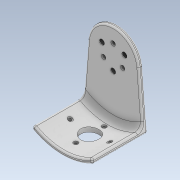
# Autodesk Inventor part: thigh_hip_connector
Saved by Autodesk Inventor 2020 (Build 240168000, 168)
## iProperties
Created: 2021-01-06
Part Number: thigh_hip_connector
Material: Generic
Document SubType Name: Modeling
Designer: DELL
Density: 1 g/cm^3
Appearance: Clear - Blue
Author: DELL
Autodesk Inventor part; units mm, degrees
ref_plane "YZ Plane" through (0, 0, 0) normal (1, 0, 0) x (0, 1, 0)
ref_plane "XZ Plane" through (0, 0, 0) normal (0, 1, 0) x (-1, 0, 0)
ref_plane "XY Plane" through (0, 0, 0) normal (0, 0, 1) x (1, 0, 0)
sketch "Sketch1" plane through (0, 0, 0) normal (0, 0, 1) x (1, 0, 0)
  circle A0 centre (0, 0) radius 22.5
  line L0 (-22.4222, 1.869) -> (-26.5, -47.0505)
  line L1 (22.4222, 1.869) -> (26.5, -47.0505)
  line L2 (9.9593, -5.75) -> (0, 0) construction
  circle A1 centre (8.4134, -4.8575) radius 2
  line L3 (0, 0) -> (9.9593, 5.75) construction
  line L4 (0, 0) -> (-9.9593, -5.75) construction
  circle A2 centre (-8.4134, -4.8575) radius 2
  circle A3 centre (0, 0) radius 9.715 construction
  circle A4 centre (0, 0) radius 11.5 construction
  circle A5 centre (0, 9.715) radius 2
  line L5 (0, 0) -> (-9.9593, 5.75) construction
  line L6 (11.5, 0) -> (-11.5, 0) construction
  circle A6 centre (-9.9593, 5.75) radius 3.75
  circle A7 centre (-9.9593, 5.75) radius 2.25
  line L7 (0, -48.5721) -> (0, 22.5) construction
  circle A8 centre (0, -11.5) radius 2.25
  circle A9 centre (0, -11.5) radius 3.75
  circle A10 centre (9.9593, 5.75) radius 3.75
  circle A11 centre (9.9593, 5.75) radius 2.25
  arc A12 (-26.1314, -42.6281) -> (26.1314, -42.6281) centre (0, 0) ccw
  arc A13 (-26.5, -47.0505) -> (26.5, -47.0505) centre (0, 0) ccw
  point P0 (0, 11.4686)
  point P1 (0, 11.4686)
  point P2 (11.5, 0)
  point P3 (-11.5, 0)
  dimension "d18" = 23
  dimension "d0" = 45
  dimension "d17" = 19.43
  dimension "d19" = 30
  dimension "d20" = 30
  dimension "d21" = 4.5
  dimension "d22" = 7.5
  dimension "d23" = 4
  dimension "d24" = 100
  dimension "d25" = 108
  dimension "d48" = 53
  constraints: 14 end point, 13 centre point, 10 coincident, 9 point on circle, 8 point on line, 6 equal radius, 2 tangent, 1 vertical, 17 other
  measures "d0" diameter of A0
  measures "d17" diameter of A3
  measures "d19" angle to the sketch x axis of L5
  measures "d20" angle to the sketch x axis of L4
  measures "d21" diameter of A11
  measures "d22" diameter of A10
  measures "d23" diameter of A5
  measures "d24" diameter of A12
  measures "d25" diameter of A13
  measures "d48" distance of L1.end L0.end
extrude "Extrusion1" add sketch "Sketch1" along normal blind 4 contours A0 | A0 L1 A12 L0 | L1 A13 L0 A12 | A1 | A2 | A5 | A6 | A9 | A10
extrude "Extrusion2" cut sketch "Sketch1" along normal blind 3.5 contours A6 | A9 | A10 | A11
extrude "Extrusion3" cut sketch "Sketch1" against normal blind 5 from surface at 4 contours A1 | A2 | A5
extrude "Extrusion4" add sketch "Sketch1" along normal blind 45 from surface at 4 contours L1 A13 L0 A12
fillet "Fillet1" radius 5 1 edges at (0, -50, 4)
fillet "Fillet2" radius 1.5 17 edges at (0, -54, 0) (0, -54, 49) (26.5, -47.0505, 24.5) (-26.5, -47.0505, 24.5) (-24.4611, -22.5907, 0) (24.4611, -22.5907, 0) (0, 22.5, 0) (-24.0409, -17.5492, 4) (-25.9834, -40.8531, 5.3489) (-26.1314, -42.6281, 29) (24.0409, -17.5492, 4) (25.9834, -40.8531, 5.3489) (26.1314, -42.6281, 29) (0, 22.5, 4) (0, -50, 49) (-26.3157, -44.8393, 49) (26.3157, -44.8393, 49)
sketch "Sketch2" plane through (0, 0, 0) normal (0, 1, 0) x (-1, 0, 0)
  circle A0 centre (0, 12) radius 2
  circle A1 centre (0, 37) radius 2
  circle A2 centre (0, 37) radius 1.25
  circle A3 centre (0, 12) radius 1.25
  line L0 (-26.3284, 0) -> (-26.3284, 49) construction
  line L1 (20.9274, 0) -> (-20.9274, 0) construction
  line L2 (24.8336, 49) -> (-24.8336, 49) construction
  line L3 (-26.3284, 24.5) -> (26.4192, 24.5) construction
  line L4 (26.4192, 47.5) -> (26.4192, 1.5) construction
  line L5 (-26.3284, 47.5) -> (-26.3284, 9) construction
  line L6 (0, 0) -> (0, 49) construction
  circle A4 centre (-17.5, 24.5) radius 1.25
  circle A5 centre (-17.5, 24.5) radius 2
  circle A6 centre (17.5, 24.5) radius 1.25
  circle A7 centre (17.5, 24.5) radius 2
  circle A8 centre (0, 24.5) radius 8
  circle A9 centre (0, 24.5) radius 25
  dimension "d30" = 4
  dimension "d31" = 2.5
  dimension "d32" = 25
  dimension "d33" = 35
  dimension "d40" = 16
  dimension "d41" = 50
  constraints: 10 centre point, 6 end point, 6 equal radius, 5 coincident, 5 point on line, 4 midpoint, 2 symmetric about line, 1 collinear, 1 vertical
  measures "d30" diameter of A1
  measures "d31" diameter of A2
  measures "d32" distance of A1.centre A0.centre
  measures "d33" distance of A6.centre A4.centre
  measures "d40" diameter of A8
  measures "d41" diameter of A9
extrude "Extrusion5" cut sketch "Sketch2" against normal through all contours A2 | A3 | A4 | A6 | A8
extrude "Extrusion6" cut sketch "Sketch2" against normal blind 51 contours A0 | A1 | A2 | A3
extrude "Extrusion7" cut sketch "Sketch2" against normal blind 47.5 contours A4 | A5 | A6 | A7
body "Solid1"
